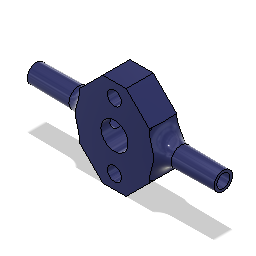
Sensor_Adapter (Autodesk Fusion 360 design; units mm, degrees)
Autodesk Fusion 360 part; units mm, degrees
sketch "Sketch1" plane through (0, 0, 0) normal (0, 0, 1) x (1, 0, 0)
  circle A0 centre (0, 0) radius 1.985
  dimension "d1" = 3.97
  measures "d1" diameter of A0
ref_plane "WorkPlane1" through (0, 0, 20) normal (0, 0, 1) x (1, 0, 0)
ref_plane "WorkPlane2" through (0, 0, 40) normal (0, 0, 1) x (1, 0, 0)
sketch "Sketch2" plane through (0, 0, 40) normal (0, 0, 1) x (1, 0, 0)
  circle A0 centre (0, 0) radius 1.985
  dimension "d7" = 3.97
  measures "d7" diameter of A0
ref_plane "WorkPlane3" through (0, 0, 27.5) normal (0, 0, 1) x (1, 0, 0)
ref_plane "WorkPlane4" through (0, 0, 12.5) normal (0, 0, 1) x (1, 0, 0)
sketch "Sketch3" plane through (0, 0, 27.5) normal (0, 0, 1) x (1, 0, 0)
  circle A0 centre (0, 0) radius 2.15
  dimension "d11" = 4.3
  measures "d11" diameter of A0
sketch "Sketch4" plane through (0, 0, 12.5) normal (0, 0, 1) x (1, 0, 0)
  circle A0 centre (0, 0) radius 2.15
  dimension "d13" = 4.3
  measures "d13" diameter of A0
loft "Loft1" add profiles "Sketch2", "Sketch3" section 1 section 2 makes body 1
loft "Loft2" add profiles "Sketch1", "Sketch4" section 1 section 2 separate body makes body 2
sketch "Sketch6" plane through (0, 0, 40) normal (0, 0, 1) x (1, 0, 0)
  circle A0 centre (0, 0) radius 1.985
  circle A1 centre (0, 0) radius 1.4
  dimension "d16" = 2.8
  measures "d16" diameter of A1
sketch "Sketch7" plane through (0, 0, 0) normal (0, 0, -1) x (-1, 0, 0)
  circle A0 centre (0, 0) radius 1.985
  circle A1 centre (0, 0) radius 1.4
  dimension "d17" = 2.8
  measures "d17" diameter of A1
extrude "Extrude1" cut sketch "Sketch6" against normal blind 10 contours A1 bodies 1
extrude "Extrude2" cut sketch "Sketch7" against normal blind 10 contours A1 bodies 2
sketch "Sketch8" plane through (0, 0, 20) normal (0, 0, 1) x (1, 0, 0)
  line L0 (2.5, -10) -> (-2.5, -10)
  line L1 (-2.5, -10) -> (-2.5, 10)
  line L2 (-2.5, 10) -> (2.5, 10)
  line L3 (2.5, 10) -> (2.5, -10)
  line L4 (2.5, -10) -> (-2.5, 10) construction
  line L5 (-2.5, -10) -> (2.5, 10) construction
  dimension "d22" = 5
  dimension "d23" = 20
extrude "Extrude3" add sketch "Sketch8" along normal mid plane 15 separate body makes body 3
combine "Combine1" operation add target body 2 tool bodies 3 1
extrude "Extrude8" cut 1 faces at (0.5498, -0.3174, 30) along direction (0, 0, -1) blind 20 on bodies 2 bodies 2
sketch "Sketch11" plane through (-2.5, 0, 0) normal (-1, 0, 0) x (0, 0, 1)
  line L0 (27.5, 10) -> (12.5, 10)
  line L1 (12.5, -10) -> (27.5, -10)
  circle A0 centre (20, 0) radius 2.9
  line L2 (27.5, -10) -> (27.5, 10)
  line L3 (12.5, 10) -> (12.5, -10)
  dimension "d42" = 5.8
  measures "d42" diameter of A0
extrude "Extrude9" cut sketch "Sketch11" against normal blind 3.6 contours A0 bodies 2
extrude "Extrude10" add 1 faces at (-2.5, 7.6306, 19.9278) along direction (-1, 0, 0) blind 0.8 on bodies 2 bodies 2
sketch "Sketch12" plane through (-3.3, 0, 0) normal (-1, 0, 0) x (0, 0, 1)
  line L0 (12.5, -10) -> (27.5, -10)
  line L1 (27.5, 10) -> (12.5, 10)
  circle A0 centre (20, 7) radius 1.5
  circle A1 centre (20, -7) radius 1.5
  circle A2 centre (20, 0) radius 2.9
  line L2 (27.5, -10) -> (27.5, 10)
  line L3 (12.5, 10) -> (12.5, -10)
  dimension "d48" = 3
  dimension "d50" = 3
  measures "d48" diameter of A0
  measures "d50" diameter of A1
extrude "Extrude11" cut sketch "Sketch12" against normal blind 2.9 contours A0 | A1 bodies 2
chamfer "Chamfer1" distance 5 angle 45 4 edges at (-0.4, 10, 27.5) (-0.4, 10, 12.5) (-0.4, -10, 12.5) (-0.4, -10, 27.5) on bodies 2
fillet "Fillet3" radius 3.5 2 edges at (-2.0045, 0.7775, 27.5) (-2.0045, 0.7775, 12.5) on bodies 2
equation "d1 = Outer_diameter_arm_end"
equation "d2 = Length_entrance_to_center"
equation "Outer_diameter_arm_end = 3.97 mm" comment "Determines the outer diamter of the piece that connects to the tubing. Original Value:3.97"
equation "Length_entrance_to_center = 20 mm" comment "This value should not be changed unless you konw what you are doing. It will mess the rest of the design up and you will have to change other values to make this work again.OV:20"
equation "d6 = Length_entrance_to_center"
equation "d7 = Outer_diameter_arm_end"
equation "Length_tubing_coverage = 12.5 mm" comment "This value should not be changed. This controls the amount of material that is initially used to create the extruding pieces coming out from the main body OV:12.5"
equation "d9 = -Length_tubing_coverage"
equation "d10 = Length_tubing_coverage"
equation "d11 = Outer_diameter_arm_start"
equation "Outer_diameter_arm_start = 4.3 mm" comment "This value dictates the OD closest to the main body. It sould be bigger than the begining of the piece so that 3D printed piece expands the tubing as it goes in.  OV:4.3"
equation "d13 = Outer_diameter_arm_start"
equation "Inner_diameter_arms = 2.8 mm" comment "This value dictates the ID of the arms extending from the main body. Should be smaller than OD. OV:2.8"
equation "d16 = Inner_diameter_arms"
equation "d17 = Inner_diameter_arms"
equation "Diameter_pressure_sensor = 5.8 mm" comment "This value dictates the diamter of the hole where the pressure sensor will fit in. OV:5.8"
equation "d42 = Diameter_pressure_sensor"
equation "Diameter_threaded_insert = 3 mm" comment "This value dictates the diameter of the hole where the threaded inserts will go in. OV:3"
equation "d48 = Diameter_threaded_insert"
equation "d50 = Diameter_threaded_insert"
